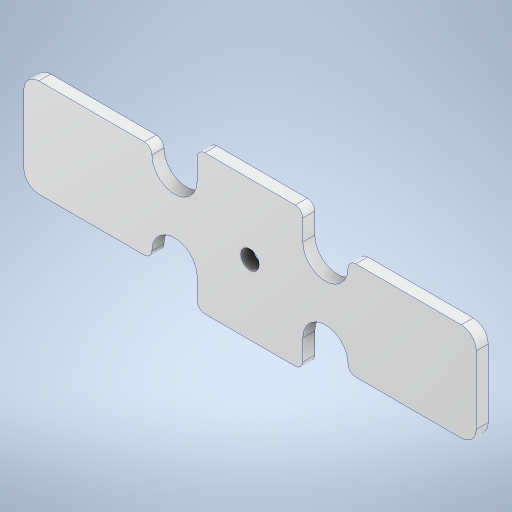
# Autodesk Inventor part: Printhead Belt Retainer Cap
Saved by Autodesk Inventor 2024 (Build 280153000, 153)
## iProperties
Created: 2025-01-04
Part Number: Printhead Belt Retainer Cap
Material: Aluminum 6061
Document SubType Name: Modeling
Designer: Ishaan
Density: 2.7 g/cm^3
Appearance: Aluminum - Flat
Author: Ishaan
Autodesk Inventor part; units mm, degrees
ref_plane "YZ Plane" through (0, 0, 0) normal (1, 0, 0) x (0, 1, 0)
ref_plane "XZ Plane" through (0, 0, 0) normal (0, 1, 0) x (-1, 0, 0)
ref_plane "XY Plane" through (0, 0, 0) normal (0, 0, 1) x (1, 0, 0)
sketch "Sketch1" plane through (0, 0, 0) normal (0, 0, 1) x (1, 0, 0)
  line L0 (13.75, -9.25) -> (-13.75, -9.25)
  line L1 (-13.75, -9.25) -> (-13.75, 9.25)
  line L2 (-13.75, 9.25) -> (13.75, 9.25)
  line L3 (13.75, 9.25) -> (13.75, -9.25)
  line L4 (13.75, -9.25) -> (-13.75, 9.25) construction
  line L5 (-13.75, -9.25) -> (13.75, 9.25) construction
  line L6 (-16, 0) -> (16, 0) construction
  circle A0 centre (-16, 0) radius 4
  circle A1 centre (16, 0) radius 4
  line L7 (30, -1) -> (-30, -1)
  line L8 (-30, -1) -> (-30, 1)
  line L9 (-30, 1) -> (30, 1)
  line L10 (30, 1) -> (30, -1)
  line L11 (30, -1) -> (-30, 1) construction
  line L12 (-30, -1) -> (30, 1) construction
  line L13 (30, -6.5) -> (-30, -6.5)
  line L14 (-30, -6.5) -> (-30, 6.5)
  line L15 (-30, 6.5) -> (30, 6.5)
  line L16 (30, 6.5) -> (30, -6.5)
  line L17 (30, -6.5) -> (-30, 6.5) construction
  line L18 (-30, -6.5) -> (30, 6.5) construction
  line L19 (10, -5.5) -> (-10, -5.5) construction
  line L20 (-10, -5.5) -> (-10, 5.5) construction
  line L21 (-10, 5.5) -> (10, 5.5) construction
  line L22 (10, 5.5) -> (10, -5.5) construction
  line L23 (10, -5.5) -> (-10, 5.5) construction
  line L24 (-10, -5.5) -> (10, 5.5) construction
  circle A2 centre (-10, 5.5) radius 3
  circle A3 centre (10, 5.5) radius 3
  circle A4 centre (10, -5.5) radius 3
  circle A5 centre (-10, -5.5) radius 3
  line L25 (7, -9.25) -> (-7, -9.25)
  line L26 (-7, -9.25) -> (-7, 9.25)
  line L27 (-7, 9.25) -> (7, 9.25)
  line L28 (7, 9.25) -> (7, -9.25)
  line L29 (7, -9.25) -> (-7, 9.25) construction
  line L30 (-7, -9.25) -> (7, 9.25) construction
  line L31 (13, -9.25) -> (-13, -9.25)
  line L32 (-13, -9.25) -> (-13, 9.25)
  line L33 (-13, 9.25) -> (13, 9.25)
  line L34 (13, 9.25) -> (13, -9.25)
  line L35 (13, -9.25) -> (-13, 9.25) construction
  line L36 (-13, -9.25) -> (13, 9.25) construction
  point P0 (0, 0)
  point P1 (-19.873, -1)
  point P2 (-13.75, -6.5)
  point P3 (13.75, -6.5)
  point P4 (19.873, -1)
  point P5 (19.873, 1)
  point P6 (13.75, 6.5)
  point P7 (-13.75, 6.5)
  point P8 (-19.873, 1)
  point P9 (-13, -6.5)
  point P10 (-13, -5.5)
  point P11 (-7, -5.5)
  point P12 (7, -5.5)
  point P13 (13, -5.5)
  point P14 (13, -6.5)
  point P15 (13, 6.5)
  point P16 (13, 5.5)
  point P17 (7, 5.5)
  point P18 (-7, 5.5)
  point P19 (-13, 5.5)
  point P20 (-13, 6.5)
  dimension "d0" = 27.5
  dimension "d1" = 18.5
  dimension "d2" = 8
  dimension "d3" = 8
  dimension "d4" = 32
  dimension "d5" = 60
  dimension "d6" = 2
  dimension "d7" = 13
  dimension "d35" = 20
  dimension "d36" = 11
  dimension "d37" = 6
  constraints: 74 end point, 13 midpoint, 12 parallel, 7 horizontal, 6 centre point, 6 coincident, 6 perpendicular, 3 equal radius, 2 point on line, 2 tangent, 1 collinear
  measures "d0" distance of L1.end L2.end
  measures "d1" distance of L0.end L1.end
  measures "d2" diameter of A0
  measures "d3" diameter of A1
  measures "d4" distance of L6.start L6.end
  measures "d5" distance of L8.end L9.end
  measures "d6" distance between parallel lines of L7 L9
  measures "d7" distance of L13.end L14.end
  measures "d35" distance of L20.end L21.end
  measures "d36" distance of L19.end L20.end
  measures "d37" diameter of A2
extrude "Extrusion1" add sketch "Sketch1" along normal blind 1.5875 contours L13 L34 A1 L3 | L3 A1 L7 L16 L13 | L0 L26 L13 L28 | A1 L34 L7 L3 | L3 L7 A1 | L13 L26 L7 L28 | A4 L28 L7 A1 L34 | L7 L34 L9 L3 | L3 L9 A1 L7 | A1 L7 L34 | A1 L9 L10 L7 | L9 L34 A1 L3 | L3 A1 L9 | L7 A1 L9 L34 | L7 L28 L9 A1 | L9 A1 L3 L15 L16 | L13 L1 A0 L32 | A5 L32 A0 L7 L26 | L7 L26 L9 L28 | A1 L34 L15 L3 | L9 A1 L34 | L9 L28 A3 L34 A1 | L13 L14 L7 A0 L1 | L7 A0 L9 L26 | L9 L26 L15 L28 | A0 L7 L1 | L1 L7 L32 A0 | L32 L7 A0 | L7 L32 L9 A0 | L9 A0 L32 A2 L26 | L7 A0 L9 L1 | L1 L9 L32 L7 | L7 L8 L9 A0 | L9 L32 A0 | L15 L26 L2 L28 | L9 A0 L1 | L1 A0 L32 L9 | L9 L14 L15 L1 A0 | A0 L1 L15 L32
fillet "Fillet2" radius 2 4 edges at (-30, 6.5, 0.7937) (-30, -6.5, 0.7937) (30, 6.5, 0.7937) (30, -6.5, 0.7937)
fillet "Fillet5" radius 1 8 edges at (-7, 9.25, 0.7937) (-7, -9.25, 0.7937) (-13, 6.5, 0.7937) (-13, -6.5, 0.7937) (13, -6.5, 0.7937) (13, 6.5, 0.7937) (7, 9.25, 0.7937) (7, -9.25, 0.7937)
sketch "Sketch3" plane through (0, 0, 1.5875) normal (0, 0, 1) x (1, 0, 0)
  point P0 (0, 0)
hole "Hole2" at (0, 0, 1.5875) direction (0, 0, -1) diameter 2.459 end through all thread size "M3x0.5" class "6H" standard "ANSI Metric M Profile"
body "Solid1"
